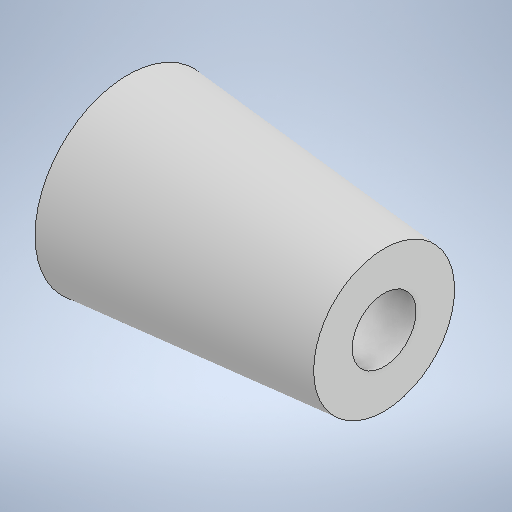
# Autodesk Inventor part: Part2
Saved by Autodesk Inventor 2025.2 (Build 292293000, 293)
## iProperties
Created: 2025-01-28
Part Number: Part2
Material: Generic
Document SubType Name: Modeling
Designer: 24oscnor
Density: 1 g/cm^3
Appearance: Default
Author: 24oscnor
Autodesk Inventor part; units mm, degrees
ref_plane "YZ Plane" through (0, 0, 0) normal (1, 0, 0) x (0, 1, 0)
ref_plane "XZ Plane" through (0, 0, 0) normal (0, 1, 0) x (-1, 0, 0)
ref_plane "XY Plane" through (0, 0, 0) normal (0, 0, 1) x (1, 0, 0)
sketch "Sketch2" plane through (0, 0, 0) normal (0, 1, 0) x (-1, 0, 0)
  line L0 (0, 14.4869) -> (20, 16.2366)
  line L1 (20, 16.2366) -> (20, 13.2252)
  line L2 (20, 13.2252) -> (0, 11.4754)
  line L3 (0, 11.4754) -> (0, 14.4869)
  line L4 (20, 8.9869) -> (0, 8.9869) construction
  point P0 (0, 0)
  dimension "d6" = 20
  dimension "d7" = 3
  dimension "d10" = 5.5
  dimension "d11" = 95
  constraints: 10 end point, 2 parallel, 1 horizontal, 1 vertical
  measures "d6" horizontal distance of L1.end L2.end
  measures "d7" distance between parallel lines of L0 L2
  measures "d10" distance from line of L0.start L4
  measures "d11" angle of L2 L1
revolve "Revolution1" add sketch "Sketch2" angle 360 about axis through (-20, 0, 8.9869) along (1, 0, 0)
body "Solid2"
